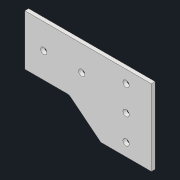
# Autodesk Inventor part: bigusset
Saved by Autodesk Inventor 2022 (Build 260153000, 153)
## iProperties
Created: 2022-09-22
Part Number: bigusset
Material: Generic
Document SubType Name: Modeling
Designer: Kieran Jarvis
Density: 1 g/cm^3
Appearance: Default
Author: Kieran Jarvis
Autodesk Inventor part; units mm, degrees
ref_plane "YZ Plane" through (0, 0, 0) normal (1, 0, 0) x (0, 1, 0)
ref_plane "XZ Plane" through (0, 0, 0) normal (0, 1, 0) x (-1, 0, 0)
ref_plane "XY Plane" through (0, 0, 0) normal (0, 0, 1) x (1, 0, 0)
sketch "Sketch1" plane through (0, 0, 0) normal (0, 0, 1) x (1, 0, 0)
  line L0 (0, 0) -> (0, 40) construction
  line L1 (0, 40) -> (-420, 40) construction
  line L2 (-420, 0) -> (-420, 40) construction
  line L3 (0, 0) -> (-420, 0) construction
  line L4 (40, 120) -> (0, 120) construction
  line L5 (0, 120) -> (0, -730) construction
  line L6 (40, -730) -> (0, -730) construction
  line L7 (40, 120) -> (40, -730) construction
  line L8 (0, 0) -> (40, 0) construction
  line L9 (40, 0) -> (40, 40) construction
  line L10 (40, 40) -> (0, 40) construction
  line L11 (0, 40) -> (0, 0) construction
  line L12 (0, 0) -> (-60, 0) construction
  line L13 (-60, 0) -> (-60, 40) construction
  line L14 (-60, 40) -> (0, 40) construction
  line L15 (0, 40) -> (0, 0) construction
  line L16 (-23.6304, 41.0957) -> (-1.8765, 58.4988) construction
  line L17 (0, 40) -> (40, 40) construction
  line L18 (40, 40) -> (40, 60) construction
  line L19 (40, 60) -> (0, 60) construction
  line L20 (0, 60) -> (0, 40) construction
  line L21 (-1.8765, 58.4988) -> (0, 60) construction
  line L22 (-23.6304, 41.0957) -> (-25, 40) construction
  line L23 (40, 0) -> (0, 0) construction
  line L24 (0, 0) -> (0, -20) construction
  line L25 (0, -20) -> (40, -20) construction
  line L26 (40, -20) -> (40, 0) construction
  line L27 (-25, 40) -> (-25, 0) construction
  line L28 (-25, 0) -> (0, -20) construction
  line L29 (20, -20) -> (20, 60) construction
  line L30 (0, 20) -> (-60, 20) construction
  line L31 (30, 10) -> (10, 10) construction
  line L32 (10, 10) -> (10, -10) construction
  line L33 (10, -10) -> (30, -10) construction
  line L34 (30, -10) -> (30, 10) construction
  line L35 (30, 10) -> (10, -10) construction
  line L36 (10, 10) -> (30, -10) construction
  line L37 (30, 30) -> (10, 30) construction
  line L38 (10, 30) -> (10, 50) construction
  line L39 (10, 50) -> (30, 50) construction
  line L40 (30, 50) -> (30, 30) construction
  line L41 (30, 30) -> (10, 50) construction
  line L42 (10, 30) -> (30, 50) construction
  line L43 (0, -20) -> (-25, 0)
  line L44 (-25, 0) -> (-60, 0)
  line L45 (-60, 0) -> (-60, 40)
  line L46 (-60, 40) -> (-25, 40)
  line L47 (-25, 40) -> (0, 60)
  line L48 (0, 60) -> (40, 60)
  line L49 (40, 60) -> (40, -20)
  line L50 (40, -20) -> (0, -20)
  line L51 (-30, 20) -> (-45, 20)
  line L52 (-30, 20) -> (-15, 20)
  point P0 (20, 0)
  point P1 (20, 0)
  point P2 (20, 40)
  point P3 (20, 30)
  point P4 (20, 10)
  point P5 (20, -10)
  dimension "d0" = 60
  dimension "d1" = 40
  dimension "d2" = 20
  dimension "d3" = 20
  dimension "d6" = 20
  dimension "d7" = 20
  dimension "d8" = 20
  dimension "d9" = 20
  dimension "d20" = 15
  dimension "d21" = 15
  constraints: 88 end point, 15 midpoint, 12 parallel, 11 perpendicular, 10 coincident, 10 point on line, 6 horizontal, 4 collinear
  measures "d0" distance of L13.end L14.end
  measures "d1" distance of L12.end L13.end
  measures "d2" distance of L18.end L17.end
  measures "d3" distance of L24.end L23.end
  measures "d6" distance of L33.end L32.end
  measures "d7" distance of L32.end L31.end
  measures "d8" distance of L38.end L39.end
  measures "d9" distance of L37.end L38.end
  measures "d20" distance of L51.start L51.end
  measures "d21" distance of L51.start L52.end
extrude "Extrusion1" add sketch "Sketch1" along normal blind 3
hole "Hole1" at (20, -10, 0) at (20, 10, 0) at (20, 30, 0) direction (0, 0, 1) diameter 5 depth 8 tip angle 118
fillet "Fillet1" radius 5 2 edges at (-25, 40, 1.5) (-25, 0, 1.5)
hole "Hole2" at (-45, 20, 0) at (-15, 20, 0) direction (0, 0, 1) diameter 5 depth 8 tip angle 118
sketch "Sketch2" plane through (0, 0, 3) normal (0, 0, 1) x (1, 0, 0)
  circle A0 centre (-45, 20) radius 2.5 projected
  circle A1 centre (-15, 20) radius 2.5 projected
  line L0 (40, -20) -> (40, 60) projected
  line L1 (40, 60) -> (0, 60) projected
  line L2 (0, 60) -> (-23.6304, 41.0957) projected
  arc A2 (-26.7539, 40) -> (-23.6304, 41.0957) centre (-26.7539, 45) ccw projected
  line L3 (-26.7539, 40) -> (-60, 40) projected
  line L4 (-60, 40) -> (-60, 0) projected
  line L5 (-60, 0) -> (-26.7539, 0) projected
  arc A3 (-23.6304, -1.0957) -> (-26.7539, 0) centre (-26.7539, -5) ccw projected
  line L6 (-23.6304, -1.0957) -> (0, -20) projected
  line L7 (0, -20) -> (40, -20) projected
  line L8 (-26.7539, 40) -> (-60, 40) projected
  line L9 (-26.7539, 40) -> (40, 40)
  point P0 (0, 0)
  constraints: 2 end point, 1 perpendicular, 1 point on line
extrude "Extrusion2" cut sketch "Sketch2" against normal blind 3 contours L9 A2 L2 L1 L0
body "Solid1"
